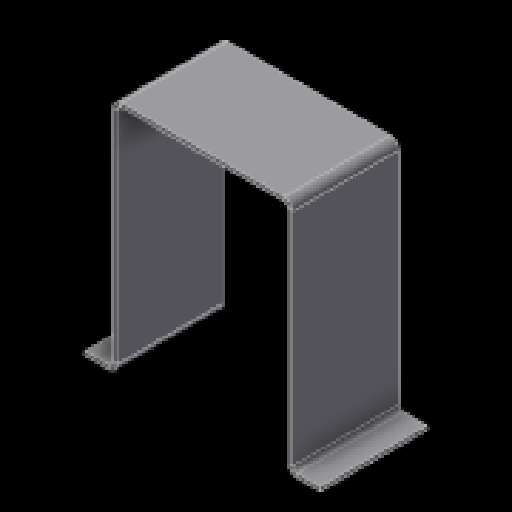
# Autodesk Inventor part: BatteryMount
Saved by Autodesk Inventor 2025.2 (Build 292293000, 293)
## iProperties
Created: 2025-11-21
Part Number: BatteryMount
Material: Generic
Document SubType Name: Sheet Metal
Designer: valer
Density: 1 g/cm^3
Sheet Metal Rule: Default
Appearance: Default
Author: valer
Autodesk Inventor part; units mm, degrees
ref_plane "YZ Plane" through (0, 0, 0) normal (1, 0, 0) x (0, 1, 0)
ref_plane "XZ Plane" through (0, 0, 0) normal (0, 1, 0) x (-1, 0, 0)
ref_plane "XY Plane" through (0, 0, 0) normal (0, 0, 1) x (1, 0, 0)
sketch "Base" plane through (0, 0, 0) normal (0, 0, 1) x (1, 0, 0)
  line L0 (161.5, 0) -> (161.5, 216)
  line L1 (161.5, 216) -> (0, 216)
  line L2 (0, 216) -> (0, 0)
  line L3 (0, 208.5) -> (0, 14)
  line L4 (-30, -5) -> (-30, 0) construction
  line L5 (161.5, 0) -> (191.5, 0)
  line L6 (0, 0) -> (-30, 0)
  line L7 (0, 0) -> (161.5, 0) construction
  line L8 (80.75, 0) -> (80.75, 216) construction
  dimension "d1" = 30
  dimension "d4" = 161.5
  dimension "d5" = 216
  measures "d1" distance of L2.end L6.end
  measures "d4" distance of L0.end L1.end
  measures "d5" distance of L0.start L0.end
contour flange "BaseFeature" sketch "Base" thickness 4 bend radius 4 width 100 along (0, 0, 1) mid plane no both sides no wall seen from (176.5, 0, 0) lies toward (0, 1, 0) curves L5 L0 L1 L2 L6
bend "Bend1"
corner "Corner1"
sketch "MountHoles" plane through (191.5, 4, 100) normal (0, 1, 0) x (1, 0, 0)
  line L0 (0, 100) -> (-22, 100) projected
  line L1 (-11, 100) -> (-11, 0) construction
  line L2 (0, 0) -> (-22, 0) projected
  line L3 (-34, 100) -> (-187.5, 100) projected
  line L4 (-110.75, 100) -> (-110.75, 0) construction
  line L5 (-34, 0) -> (-187.5, 0) projected
  circle A0 centre (-11, 90) radius 3
  line L6 (0, 100) -> (0, 0) projected
  line L7 (0, 50) -> (-11, 50) construction
  circle A1 centre (-11, 10) radius 3
  circle A2 centre (-210.5, 90) radius 3
  circle A3 centre (-210.5, 10) radius 3
  point P0 (-191.5, 100)
  dimension "d17" = 6
  dimension "d18" = 10
  constraints: 6 end point, 6 midpoint, 4 centre point, 3 symmetric about line, 1 point on line, 3 other
  measures "d17" diameter of A0
  measures "d18" distance from line of L0 A0.centre
extrude "MountHolesFeature" cut sketch "MountHoles" against normal blind 4
fillet "FilletsFeature" radius 6 4 edges at (191.5, 2, 0) (191.5, 2, 100) (-30, 2, 0) (-30, 2, 100)
equation "\"d19\" = Thickness"
equation "\"d6\" = Thickness"
equation "\"d7\" = BendReliefWidth"
equation "\"d8\" = BendReliefDepth"
equation "\"d9\" = MinimumRemnant"
equation "\"d10\" = TransitionRadius"
equation "\"d12\" = BendRadius"
equation "\"d14\" = CornerReliefSize"
equation "\"d15\" = GapSize"
equation "\"d16\" = JacobiRadiusSize"
equation "\"BendRadius\" = Thickness"
equation "\"BendReliefWidth\" = Thickness"
equation "\"BendReliefDepth\" = 0.5 * Thickness"
equation "\"CornerReliefSize\" = 4 * Thickness"
equation "\"MinimumRemnant\" = 2 * Thickness"
equation "\"TransitionRadius\" = BendRadius"
equation "\"JacobiRadiusSize\" = BendRadius"
equation "\"GapSize\" = Thickness"
equation "\"Thickness\" = 4"
body "Solid1"
